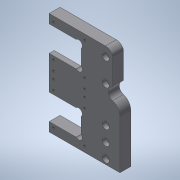
# Autodesk Inventor part: Zlifter
Saved by Autodesk Inventor 2020 (Build 240168000, 168)
## iProperties
Created: 2019-05-25
Part Number: Zlifter
Material: Generic
Document SubType Name: Modeling
Designer: LillaHunden
Density: 1 g/cm^3
Appearance: Default
Author: LillaHunden
Autodesk Inventor part; units mm, degrees
ref_plane "YZ Plane" through (0, 0, 0) normal (1, 0, 0) x (0, 1, 0)
ref_plane "XZ Plane" through (0, 0, 0) normal (0, 1, 0) x (-1, 0, 0)
sketch "Sketch1" plane through (0, 0, 0) normal (0, 0, 1) x (1, 0, 0)
  circle A0 centre (-14.5473, 15.1065) radius 1.65 construction
  circle A1 centre (16.4527, 46.1065) radius 1.65 construction
  circle A2 centre (-14.5473, 46.1065) radius 1.65 construction
  circle A3 centre (16.4527, 15.1065) radius 1.65 construction
  circle A4 centre (0.5246, -13.3925) radius 6.1 construction
  circle A5 centre (0.9527, 30.6065) radius 4.765 construction
  circle A6 centre (-32.0049, -58.1419) radius 2.2 construction
  circle A7 centre (-32.0049, -26.1419) radius 2.2 construction
  circle A8 centre (-21.0049, -26.1419) radius 2.2 construction
  circle A9 centre (-32.0049, -42.1419) radius 2.2 construction
  circle A10 centre (-32.0049, 13.8581) radius 2.2 construction
  arc A11 (27.3227, 8.6665) -> (21.7227, 8.6665) centre (24.5227, 8.6665) ccw construction
  line L0 (27.3227, 8.6665) -> (27.3227, 5.6665) construction
  arc A12 (21.7227, 5.6665) -> (27.3227, 5.6665) centre (24.5227, 5.6665) ccw construction
  line L1 (21.7227, 5.6665) -> (21.7227, 8.6665) construction
  arc A13 (-19.8173, 8.6665) -> (-25.4173, 8.6665) centre (-22.6173, 8.6665) ccw construction
  line L2 (-19.8173, 8.6665) -> (-19.8173, 5.6665) construction
  arc A14 (-25.4173, 5.6665) -> (-19.8173, 5.6665) centre (-22.6173, 5.6665) ccw construction
  line L3 (-25.4173, 5.6665) -> (-25.4173, 8.6665) construction
  arc A15 (27.3227, 55.8065) -> (21.7227, 55.8065) centre (24.5227, 55.8065) ccw construction
  line L4 (27.3227, 55.8065) -> (27.3227, 52.8065) construction
  arc A16 (21.7227, 52.8065) -> (27.3227, 52.8065) centre (24.5227, 52.8065) ccw construction
  line L5 (21.7227, 52.8065) -> (21.7227, 55.8065) construction
  arc A17 (-25.4173, 52.8065) -> (-19.8173, 52.8065) centre (-22.6173, 52.8065) ccw construction
  line L6 (-25.4173, 52.8065) -> (-25.4173, 55.8065) construction
  arc A18 (-19.8173, 55.8065) -> (-25.4173, 55.8065) centre (-22.6173, 55.8065) ccw construction
  line L7 (-19.8173, 55.8065) -> (-19.8173, 52.8065) construction
  arc A19 (36.0049, 57.8065) -> (30.0049, 63.8065) centre (30.0049, 57.8065) ccw construction
  line L8 (30.0049, 63.8065) -> (-34.0049, 63.8065) construction
  arc A20 (-34.0049, 63.8065) -> (-40.0049, 57.8065) centre (-34.0049, 57.8065) ccw construction
  line L9 (-40.0049, -59.8065) -> (-40.0049, 57.8065) construction
  arc A21 (-40.0049, -59.8065) -> (-36.0049, -63.8065) centre (-36.0049, -59.8065) ccw construction
  line L10 (-19.1877, -63.8065) -> (-36.0049, -63.8065) construction
  arc A22 (-19.1877, -63.8065) -> (-12.1142, -59.5435) centre (-19.1877, -55.8065) ccw construction
  arc A23 (33.0556, -4.4538) -> (-12.1142, -59.5435) centre (145.8325, -142.9862) ccw construction
  arc A24 (33.0556, -4.4538) -> (36.0049, 1.7503) centre (28.0049, 1.7503) ccw construction
  line L11 (36.0049, 1.7503) -> (36.0049, 57.8065) construction
  line L12 (-36.0049, -63.8065) -> (-30.0709, -63.8065)
  line L13 (-40.0049, 38.1885) -> (-40.0049, -59.8065)
  line L14 (-26.0709, -19.8799) -> (-18.1973, -19.8799)
  line L15 (-16.1973, -21.8799) -> (-16.1973, -30.4039)
  line L16 (-18.1973, -32.4039) -> (-26.0709, -32.4039)
  line L17 (-40.0049, -31.0336) -> (-40.0049, -21.6758)
  line L18 (-28.0709, -61.8065) -> (-28.0709, -34.4039)
  line L19 (-28.0709, -17.8799) -> (-28.0709, 38.9681)
  arc A25 (-16.1973, -21.8799) -> (-18.1973, -19.8799) centre (-18.1973, -21.8799) ccw
  arc A26 (-18.1973, -32.4039) -> (-16.1973, -30.4039) centre (-18.1973, -30.4039) ccw
  arc A27 (-26.0709, -32.4039) -> (-28.0709, -34.4039) centre (-26.0709, -34.4039) ccw
  arc A28 (-28.0709, -17.8799) -> (-26.0709, -19.8799) centre (-26.0709, -17.8799) ccw
  arc A29 (-30.0709, -63.8065) -> (-28.0709, -61.8065) centre (-30.0709, -61.8065) ccw
  line L20 (-34.0379, -63.8065) -> (-40.0049, -63.8065)
  line L21 (-40.0049, -63.8065) -> (-40.0049, -59.8065)
  line L22 (-28.0709, 24.8307) -> (-28.0709, 49.4852)
  line L23 (-28.0709, 49.4852) -> (-40.0049, 49.4852)
  line L24 (-40.0049, 49.4852) -> (-40.0049, 24.8307)
  line L25 (-40.0049, 49.4852) -> (-94.362, 49.4852)
  line L26 (-94.362, 49.4852) -> (-94.362, -63.8065)
  line L27 (-94.362, -63.8065) -> (-40.0049, -63.8065)
  line L28 (-40.0049, -63.8065) -> (-40.0049, 49.4852)
  circle A30 centre (-32.0049, 39.5529) radius 2.2 projected
  line L29 (-28.0709, -61.8065) -> (-28.0709, -63.8065)
  line L30 (-30.0709, -63.8065) -> (-28.0709, -63.8065)
  point P0 (0, 0)
  point P1 (-16.1973, -26.1419)
  dimension "d0" = 2
  dimension "d1" = 2
  constraints: 38 end point, 13 tangent, 12 point on circle, 7 parallel, 6 perpendicular, 6 point on line, 5 centre point, 3 equal radius, 3 horizontal, 1 collinear, 1 horizontal alignment, 1 midpoint
  measures "d0" radius of A25
  measures "d1" radius of A29
extrude "Extrusion1" add sketch "Sketch1" along normal blind 12 contours L20 L21 L13 L24 L23 L22 L19 A28 L14 A25 L15 A26 L16 A27 L18 A29 L12 | L27 L26 L25 L24 L13 L21 | A29 L29 L30 | A30
sketch "Sketch6" plane through (0, 0, 12) normal (0, 0, 1) x (1, 0, 0)
  circle A0 centre (-62.3466, 14.8452) radius 1.621 construction
  circle A1 centre (-89.4766, 36.7552) radius 1.621 construction
  circle A2 centre (-88.9966, 14.8652) radius 1.621 construction
  circle A3 centre (-62.5266, 36.1352) radius 1.621 construction
  line L0 (-59.0466, 11.4852) -> (-92.9766, 11.4852) construction
  line L1 (-59.0466, 39.4852) -> (-59.0466, 11.4852) construction
  line L2 (-92.9766, 39.4852) -> (-59.0466, 39.4852) construction
  line L3 (-92.9766, 11.4852) -> (-92.9766, 39.4852) construction
  circle A4 centre (-89.7266, -29.1665) radius 1.621 construction
  circle A5 centre (-62.5966, -51.0765) radius 1.621 construction
  circle A6 centre (-63.0766, -29.1865) radius 1.621 construction
  circle A7 centre (-89.5466, -50.4565) radius 1.621 construction
  line L4 (-93.0266, -25.8065) -> (-59.0966, -25.8065) construction
  line L5 (-93.0266, -53.8065) -> (-93.0266, -25.8065) construction
  line L6 (-59.0966, -53.8065) -> (-93.0266, -53.8065) construction
  line L7 (-59.0966, -25.8065) -> (-59.0966, -53.8065) construction
  line L8 (-58.9466, 39.5852) -> (-58.9466, 11.3852)
  line L9 (-58.9466, 11.3852) -> (-93.0766, 11.3852)
  line L10 (-93.0766, 11.3852) -> (-93.0766, 39.5852)
  line L11 (-93.0766, 39.5852) -> (-58.9466, 39.5852)
  line L12 (-58.9966, -25.7065) -> (-93.1266, -25.7065)
  line L13 (-93.1266, -25.7065) -> (-93.1266, -53.9065)
  line L14 (-93.1266, -53.9065) -> (-58.9966, -53.9065)
  line L15 (-58.9966, -53.9065) -> (-58.9966, -25.7065)
  line L16 (-58.9466, 11.3852) -> (-62.3466, 14.8452) construction
  circle A8 centre (-61.7502, 14.2383) radius 4
  circle A9 centre (-61.7751, 36.7568) radius 4
  line L17 (-58.9466, 39.5852) -> (-65.6626, 32.8692) construction
  line L18 (-94.362, 49.4852) -> (-94.362, -63.8065) projected
  line L19 (-93.0766, 39.5852) -> (-94.362, 39.5852)
  line L20 (-94.362, 39.5852) -> (-94.362, 11.4346)
  line L21 (-94.362, 11.4346) -> (-93.0766, 11.4346)
  line L22 (-93.0766, 11.4346) -> (-93.0766, 39.5852)
  point P0 (0, 0)
  point P1 (-64.5538, 11.3852)
  point P2 (-58.9466, 17.0913)
  point P3 (-58.9466, 33.9284)
  point P4 (-64.6035, 39.5852)
  point P5 (-94.362, 39.5852)
  point P6 (-94.362, 39.5852)
  dimension "d19" = 8
  dimension "d20" = 8
  dimension "d16" = 0.1
  dimension "d17" = 0.1
  dimension "d21" = 45
  constraints: 28 end point, 3 point on line, 2 parallel, 1 horizontal, 1 perpendicular, 12 other
  measures "d16" distance between parallel lines of L2 L11
  measures "d17" distance between parallel lines of L4 L12
  measures "d21" angle of L8 L17
extrude "Extrusion6" cut sketch "Sketch6" against normal through all contours A9 L8 | L8 A9 L11 | L11 A9 | L8 A8 L9 L10 L11 A9 | A8 L8 | L8 L9 A8 | A8 L9
sketch "Sketch7" plane through (0, 0, 12) normal (0, 0, 1) x (1, 0, 0)
  circle A0 centre (-89.7266, -29.1665) radius 1.621 construction
  circle A1 centre (-62.5966, -51.0765) radius 1.621 construction
  circle A2 centre (-63.0766, -29.1865) radius 1.621 construction
  circle A3 centre (-89.5466, -50.4565) radius 1.621 construction
  line L0 (-93.0266, -25.8065) -> (-59.0966, -25.8065) construction
  line L1 (-93.0266, -53.8065) -> (-93.0266, -25.8065) construction
  line L2 (-59.0966, -53.8065) -> (-93.0266, -53.8065) construction
  line L3 (-59.0966, -25.8065) -> (-59.0966, -53.8065) construction
  line L4 (-58.9966, -25.7065) -> (-93.1266, -25.7065)
  line L5 (-93.1266, -25.7065) -> (-93.1266, -53.9065)
  line L6 (-93.1266, -53.9065) -> (-58.9966, -53.9065)
  line L7 (-58.9966, -53.9065) -> (-58.9966, -25.7065)
  line L8 (-58.9966, -25.7065) -> (-69.2955, -36.0054) construction
  line L9 (-58.9966, -53.9065) -> (-69.6417, -43.2615) construction
  circle A4 centre (-61.8251, -28.535) radius 4
  circle A5 centre (-61.8251, -51.0781) radius 4
  line L10 (-94.362, 49.4852) -> (-94.362, -63.8065) projected
  line L11 (-93.1266, -25.7065) -> (-94.362, -25.7065)
  line L12 (-94.362, -25.7065) -> (-94.362, -53.9065)
  line L13 (-94.362, -53.9065) -> (-93.1266, -53.9065)
  line L14 (-93.1266, -53.9065) -> (-93.1266, -25.7065)
  point P0 (0, 0)
  point P1 (-94.362, 11.4346)
  point P2 (-58.9966, -48.2497)
  point P3 (-58.9966, -31.3634)
  point P4 (-64.6535, -25.7065)
  point P5 (-64.6535, -53.9065)
  dimension "d27" = 8
  dimension "d28" = 8
  dimension "d24" = 0.1
  dimension "d25" = 45
  dimension "d26" = 45
  constraints: 20 end point, 3 point on line, 2 parallel, 1 horizontal, 1 perpendicular, 9 other
  measures "d24" distance between parallel lines of L0 L4
  measures "d25" angle of L7 L9
  measures "d26" angle of L7 L8
extrude "Extrusion7" cut sketch "Sketch7" against normal through all
sketch "Sketch8" plane through (0, 0, 12) normal (0, 0, 1) x (1, 0, 0)
  point P0 (-55.0966, 43.4852)
  point P1 (-89.4766, 43.4852)
  point P2 (-55.0966, 7.4852)
  point P3 (-89.4766, 7.4852)
  point P4 (-89.4766, -21.8065)
  point P5 (-55.0966, -21.8065)
  point P6 (-55.0966, -57.8065)
  point P7 (-89.4766, -57.8065)
  point P8 (-89.4766, -3.1607)
  point P9 (-55.0966, -3.1607)
  point P10 (-55.0966, -11.1607)
  point P11 (-89.4766, -11.1607)
hole "Hole1" at (-55.0966, 43.4852, 12) at (-89.4766, 43.4852, 12) at (-55.0966, 7.4852, 12) at (-89.4766, 7.4852, 12) at (-89.4766, -21.8065, 12) at (-55.0966, -21.8065, 12) at (-55.0966, -57.8065, 12) at (-89.4766, -57.8065, 12) at (-89.4766, -3.1607, 12) at (-55.0966, -3.1607, 12) at (-55.0966, -11.1607, 12) at (-89.4766, -11.1607, 12) direction (0, 0, -1) diameter 2.459 depth 8.4 tip angle 120 thread size "M3x0.5" class "6H" standard "ISO Metric profile"
sketch "Sketch9" plane through (0, 0, 12) normal (0, 0, 1) x (1, 0, 0)
  point P0 (-21.0049, -26.1419)
  point P1 (-32.0049, -26.1419)
  point P2 (-32.0049, -42.1419)
  point P3 (-32.0049, -58.1419)
  point P4 (-32.0049, 13.8581)
hole "Hole3" at (-21.0049, -26.1419, 12) at (-32.0049, -26.1419, 12) at (-32.0049, -42.1419, 12) at (-32.0049, -58.1419, 12) at (-32.0049, 13.8581, 12) direction (0, 0, -1) diameter 4.8 depth 12 counterbore diameter 8 counterbore depth 4.5
sketch "Sketch10" plane through (0, 0, 12) normal (0, 0, 1) x (1, 0, 0)
  point P0 (-32.0049, 39.5529)
hole "Hole5" at (-32.0049, 39.5529, 12) direction (0, 0, -1) diameter 4.5 depth 12 counterbore diameter 8 counterbore depth 4.5
sketch "Sketch11" plane through (0, 0, 12) normal (0, 0, 1) x (1, 0, 0)
  line L0 (-28.0709, 49.4852) -> (-94.362, 49.4852) projected
  line L1 (-28.0709, 49.4852) -> (-16.1973, 49.4852)
  line L2 (-16.1973, 49.4852) -> (-16.1973, -63.8065)
  line L3 (-16.1973, -63.8065) -> (-28.0709, -63.8065)
  line L4 (-28.0709, -63.8065) -> (-28.0709, 49.4852)
  line L5 (-16.1973, -30.4039) -> (-16.1973, -21.8799) projected
  point P0 (0, 0)
  point P1 (-30.0709, -63.8065)
  point P2 (-16.1973, -26.1419)
  constraints: 8 end point, 2 parallel, 1 horizontal, 1 horizontal alignment, 1 midpoint, 1 perpendicular, 1 point on line
ref_plane "Work Plane1" through (-40.0049, -63.8065, 0) normal (0, 0, 1) x (1, 0, 0)
extrude "Extrusion8" add sketch "Sketch11" against normal up to surface (12 mm away)
sketch "Sketch12" plane through (0, 0, 12) normal (0, 0, 1) x (1, 0, 0)
  circle A0 centre (-22.6173, 7.0365) radius 5 construction
  circle A1 centre (-22.6173, 7.0365) radius 6.2937
  line L0 (-16.1973, -63.8065) -> (-16.1973, 49.4852) construction
  arc A2 (-16.1973, -9.7731) -> (-24.3719, 0.9924) centre (-27.5322, -9.8937) ccw
  line L1 (-22.6173, 7.0365) -> (-6.8472, 7.0365) construction
  arc A3 (-24.3719, 13.0807) -> (-16.1973, 23.8461) centre (-27.5322, 23.9668) ccw
  line L2 (-16.1973, 23.8461) -> (-16.1973, -9.7731)
  point P0 (0, 0)
  point P1 (-24.3719, 13.0807)
  constraints: 4 end point, 4 point on circle, 3 symmetric about line, 2 centre point, 1 collinear, 1 horizontal, 1 point on line, 5 other
extrude "Extrusion9" cut sketch "Sketch12" against normal through all
sketch "Sketch13" plane through (0, 0, 12) normal (0, 0, 1) x (1, 0, 0)
  line L0 (-93.0766, 11.3852) -> (-93.0766, 39.5852) projected
  line L1 (-93.0766, 39.5852) -> (-64.6035, 39.5852) projected
  line L2 (-64.5538, 11.3852) -> (-93.0766, 11.3852) projected
  line L3 (-93.0766, 39.5852) -> (-94.5692, 39.5852)
  line L4 (-94.5692, 39.5852) -> (-94.5692, 11.3852)
  line L5 (-94.5692, 11.3852) -> (-93.0766, 11.3852)
  line L6 (-93.0766, 11.3852) -> (-93.0766, 39.5852)
  point P0 (0, 0)
  constraints: 8 end point, 2 parallel, 1 horizontal, 1 perpendicular
extrude "Extrusion10" cut sketch "Sketch13" against normal through all
fillet "Fillet2" radius 5.25 1 edges at (-16.1973, 49.4852, 6)
sketch "Sketch14" plane through (-94.362, 11.3852, 0) normal (-1, 0, 0) x (0, 0, 1)
  line L0 (3.6, -31.9623) -> (12, -31.9623) projected
  line L1 (6.5397, -31.9623) -> (-1.0136, -31.9623)
  line L2 (-1.0136, -31.9623) -> (-1.0136, -37.4571)
  line L3 (-1.0136, -37.4571) -> (6.5397, -37.4571)
  line L4 (6.5397, -37.4571) -> (6.5397, -31.9623)
  point P0 (0, -11.3852)
  constraints: 8 end point, 2 parallel, 1 horizontal, 1 perpendicular, 1 point on line
extrude "Extrusion11" cut sketch "Sketch14" against normal blind 33.25
sketch "Sketch15" plane through (-94.362, 11.3852, 0) normal (-1, 0, 0) x (0, 0, 1)
  line L0 (6.5397, -37.0918) -> (12, -37.0918) projected
  line L1 (0, 0) -> (0, -31.9623) projected
  line L2 (6.5397, -37.0918) -> (0, -37.0918)
  line L3 (0, -37.0918) -> (0, 0)
  line L4 (0, 0) -> (6.5397, 0)
  line L5 (6.5397, 0) -> (6.5397, -37.0918)
  point P0 (0, -11.3852)
  constraints: 8 end point, 2 parallel, 2 point on line, 1 horizontal, 1 perpendicular
extrude "Extrusion12" cut sketch "Sketch15" against normal up to surface (35.4154 mm away)
sketch "Sketch16" plane through (0, 0, 12) normal (0, 0, 1) x (1, 0, 0)
  line L0 (-21.4473, 49.4852) -> (-94.362, 49.4852) projected
  arc A0 (-24.3719, 44.3279) -> (-32.2042, 49.4852) centre (-32.2042, 40.9593) ccw
  line L1 (-24.3719, 44.3279) -> (-24.3719, 14.0261)
  arc A1 (-24.3719, 13.0807) -> (-24.3719, 0.9924) centre (-22.6173, 7.0365) ccw projected
  arc A2 (-24.3719, 14.0261) -> (-28.902, 7.3725) centre (-21.1413, 6.9576) ccw
  arc A3 (-24.3719, 13.0807) -> (-24.3719, 0.9924) centre (-22.6173, 7.0365) ccw projected
  arc A4 (-28.0709, -41.4187) -> (-28.0709, -42.8651) centre (-32.0049, -42.1419) ccw projected
  line L2 (-28.0709, -41.4187) -> (-28.0709, -42.8651) projected
  line L3 (-28.0709, -57.4187) -> (-28.0709, -58.8651) projected
  arc A5 (-28.0709, -57.4187) -> (-28.0709, -58.8651) centre (-32.0049, -58.1419) ccw projected
  arc A6 (-28.0709, 14.5813) -> (-28.0709, 13.1349) centre (-32.0049, 13.8581) ccw projected
  line L4 (-28.0709, 14.5813) -> (-28.0709, 13.1349) projected
  arc A7 (-28.0709, -25.4187) -> (-28.0709, -26.8651) centre (-32.0049, -26.1419) ccw projected
  line L5 (-28.0709, -25.4187) -> (-28.0709, -26.8651) projected
  circle A8 centre (-55.0966, -11.1607) radius 1.2295 projected
  circle A9 centre (-89.4766, -3.1607) radius 1.2295 projected
  circle A10 centre (-55.0966, -57.8065) radius 1.2295 projected
  circle A11 centre (-89.4766, -21.8065) radius 1.2295 projected
  circle A12 centre (-55.0966, 7.4852) radius 1.2295 projected
  circle A13 centre (-55.0966, 43.4852) radius 1.2295 projected
  circle A14 centre (-89.4766, 43.4852) radius 1.2295 projected
  circle A15 centre (-89.4766, 7.4852) radius 1.2295 projected
  circle A16 centre (-55.0966, -21.8065) radius 1.2295 projected
  circle A17 centre (-89.4766, -57.8065) radius 1.2295 projected
  circle A18 centre (-55.0966, -3.1607) radius 1.2295 projected
  circle A19 centre (-89.4766, -11.1607) radius 1.2295 projected
  line L6 (-28.0709, 40.2761) -> (-28.0709, 38.8298) projected
  arc A20 (-28.0709, 40.2761) -> (-28.0709, 38.8298) centre (-32.0049, 39.5529) ccw projected
  arc A21 (-16.1973, 44.2352) -> (-21.4473, 49.4852) centre (-21.4473, 44.2352) ccw projected
  line L7 (-21.4473, 49.4852) -> (-94.362, 49.4852) projected
  line L8 (-94.362, 49.4852) -> (-94.362, 39.5852) projected
  line L9 (-94.362, 39.5852) -> (-64.6035, 39.5852) projected
  arc A22 (-58.9466, 33.9284) -> (-64.6035, 39.5852) centre (-61.7751, 36.7568) ccw projected
  line L10 (-58.9466, 33.9284) -> (-58.9466, 17.0913) projected
  arc A23 (-64.5538, 11.3852) -> (-58.9466, 17.0913) centre (-61.7502, 14.2383) ccw projected
  line L11 (-64.5538, 11.3852) -> (-94.362, 11.3852) projected
  line L12 (-94.362, 11.3852) -> (-94.362, -25.7065) projected
  line L13 (-94.362, -25.7065) -> (-64.6535, -25.7065) projected
  arc A24 (-58.9966, -31.3634) -> (-64.6535, -25.7065) centre (-61.8251, -28.535) ccw projected
  line L14 (-58.9966, -31.3634) -> (-58.9966, -48.2497) projected
  arc A25 (-64.6535, -53.9065) -> (-58.9966, -48.2497) centre (-61.8251, -51.0781) ccw projected
  line L15 (-64.6535, -53.9065) -> (-94.362, -53.9065) projected
  line L16 (-94.362, -53.9065) -> (-94.362, -63.8065) projected
  line L17 (-94.362, -63.8065) -> (-16.1973, -63.8065) projected
  line L18 (-16.1973, -63.8065) -> (-16.1973, -9.7731) projected
  arc A26 (-16.1973, -9.7731) -> (-24.3719, 0.9924) centre (-27.5322, -9.8937) ccw projected
  arc A27 (-24.3719, 13.0807) -> (-24.3719, 0.9924) centre (-22.6173, 7.0365) ccw projected
  arc A28 (-24.3719, 13.0807) -> (-16.1973, 23.8461) centre (-27.5322, 23.9668) ccw projected
  line L19 (-16.1973, 23.8461) -> (-16.1973, 44.2352) projected
  point P0 (0, 0)
  point P1 (-24.3719, 13.0807)
  constraints: 5 point on circle, 2 centre point, 2 end point, 2 tangent, 1 point on line, 1 vertical
extrude "Extrusion13" cut sketch "Sketch16" against normal through all contours A21 L19 A28 A1 A2 L1 A0 L0
fillet "Fillet3" radius 4 1 edges at (-24.3719, 44.3279, 6)
fillet "Fillet4" radius 2 1 edges at (-24.3719, 14.0261, 6)
body "Solid1"
